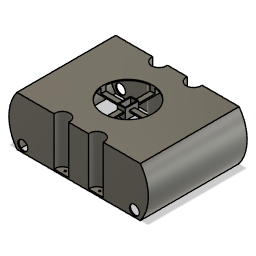
Carter (Autodesk Fusion 360 design; units mm, degrees)
Autodesk Fusion 360 part; units mm, degrees
sketch "Sketch1" plane through (0, 0, 0) normal (0, 0, 1) x (1, 0, 0)
  line L0 (0, 0) -> (-125, 0)
  line L1 (-125, 100) -> (0, 100)
  line L2 (0, 100) -> (0, 0)
  arc A0 (-125, 100) -> (-125, 0) centre (-56.2614, 50) ccw
  arc A1 (-124.4112, 98) -> (-123, 0) centre (-54.2614, 50) ccw
  line L3 (0, 98) -> (-124.4112, 98)
  line L4 (-175, 98) -> (-175, -10)
  line L5 (-175, -10) -> (191.1619, -10)
  line L6 (191.1619, -10) -> (191.1619, 126.0853)
  line L7 (191.1619, 126.0853) -> (-175, 126.0853)
  line L8 (-175, 126.0853) -> (-175, 98)
  line L9 (0, 98) -> (124.4112, 98)
  line L10 (125, 100) -> (0, 100)
  arc A2 (123, 0) -> (124.4112, 98) centre (54.2614, 50) ccw
  arc A3 (125, 0) -> (125, 100) centre (56.2614, 50) ccw
  line L11 (0, 0) -> (125, 0)
  circle A4 centre (113, 12.5) radius 10
  circle A5 centre (-113, 12.5) radius 10
  dimension "d1" = 125
  dimension "d2" = 100
  dimension "d3" = 85
  dimension "d4" = 85
  dimension "d6" = 2
  dimension "d7" = 2
  dimension "d44" = 20
  dimension "d45" = 12
  dimension "d46" = 12.5
  constraint horizontal L0
  constraint horizontal L1
  constraint vertical L2
  constraint coincident L0.start L2.end
  constraint coincident L0 A1.end
  constraint coincident L2 L3.start
  constraint perpendicular L2 L3
  constraint perpendicular L3 L4
  constraint perpendicular L4 L5
  constraint perpendicular L5 L6
  constraint perpendicular L6 L7
  constraint perpendicular L3 L8
  constraint symmetric L0.start L2 L11.start
  constraint symmetric L0.end L2 A3.start
  constraint symmetric L1.start L2 L10.start
  constraint symmetric L1.end L2 L10.end
  constraint symmetric L2 A0 A3
  constraint symmetric L2 A1.end A2.start
  constraint symmetric L2 A1 A2
  constraint symmetric L2 L3.start L9.start
  constraint symmetric L2 A1.start L9.end
  constraint symmetric L2 A4 A5
  measures "d1" distance of L0.start L0.end
  measures "d2" distance of L0.start L1.end
  measures "d3" radius of A0
  measures "d4" radius of A1
  measures "d6" distance of L0.end A1.end
  measures "d7" distance of L1 L3
  measures "d44" diameter of A4
  measures "d45" horizontal distance of A3.start A4.centre
  measures "d46" distance of L11 A4.centre
extrude "Extrude1" add sketch "Sketch1" along normal blind 196 contours L0 L1 L2 A0 A1 L3 | L2 L9 L10 A2 A3 L11 makes body 1
sketch "Sketch2" plane through (0, 100, 0) normal (0, 1, 0) x (-1, 0, 0)
  line L0 (-125, 0) -> (125, 0)
  line L1 (125, 0) -> (125, 196)
  line L2 (125, 196) -> (-125, 196)
  line L3 (-125, 196) -> (-125, 0)
  line L4 (56.5763, 0) -> (165.4437, 0)
  line L5 (165.4437, 0) -> (165.4437, -2)
  line L6 (165.4437, -2) -> (56.5763, -2)
  line L7 (56.5763, -2.1497) -> (56.5763, -2)
  line L8 (27.1632, 196) -> (155, 196)
  line L9 (155, 196) -> (155, 198)
  line L10 (155, 198) -> (27.1632, 198)
  line L11 (27.1632, 196) -> (-160, 196)
  line L12 (-160, 196) -> (-160, 198)
  line L13 (-160, 198) -> (27.1632, 198)
  line L14 (56.5763, 0) -> (-160, 0)
  line L15 (-160, 0) -> (-160, -2)
  line L16 (-160, -2) -> (56.5763, -2)
  line L17 (56.5763, -2) -> (56.5763, 0)
  circle A0 centre (-35, 196) radius 15
  circle A1 centre (-35, 196) radius 17
  circle A2 centre (35, 196) radius 15
  circle A3 centre (35, 196) radius 17
  circle A4 centre (-35, 0) radius 17
  circle A5 centre (-35, 0) radius 15
  circle A6 centre (35, 0) radius 17
  circle A7 centre (35, 0) radius 15
  circle A8 centre (-35, 6) radius 2
  circle A9 centre (35, 6) radius 2
  line L18 (-50, 0) -> (-50, 25)
  line L19 (20, 0) -> (20, 24.2158)
  circle A10 centre (35, 190) radius 2
  circle A11 centre (-35, 190) radius 2
  circle A12 centre (0, 98) radius 50
  line L20 (65, 103) -> (65, 93)
  line L21 (-65, 93) -> (-65, 103)
  line L22 (-5, 33) -> (5, 33)
  line L23 (5, 163) -> (-5, 163)
  line L24 (-6, 109.5) -> (6, 109.5)
  line L25 (6, 86.5) -> (-6, 86.5)
  line L26 (-8, 93) -> (-65, 93)
  line L27 (65, 93) -> (8, 93)
  line L28 (5, 33) -> (5, 84.5)
  line L29 (5, 111.5) -> (5, 163)
  line L30 (65, 103) -> (8, 98.6154) construction
  line L31 (-8, 97.3846) -> (-65, 93) construction
  line L32 (-65, 103) -> (-8, 98.6154) construction
  line L33 (8, 97.3846) -> (65, 93) construction
  line L34 (-125, 98) -> (-8, 98)
  line L35 (8, 98) -> (125, 98)
  line L36 (-5, 33) -> (-1.0385, 84.5) construction
  line L37 (1.0385, 111.5) -> (5, 163) construction
  line L38 (5, 33) -> (1.0385, 84.5) construction
  line L39 (-1.0385, 111.5) -> (-5, 163) construction
  line L40 (-65, 103) -> (-8, 103)
  line L41 (8, 103) -> (65, 103)
  line L42 (-5, 84.5) -> (-5, 33)
  line L43 (-5, 163) -> (-5, 111.5)
  line L44 (6, 109.5) -> (6, 98)
  line L45 (6, 97.5385) -> (6, 86.5)
  line L46 (-6, 86.5) -> (-6, 98.4615)
  line L47 (-6, 103) -> (-6, 109.5)
  line L48 (-6, 103) -> (-6, 98.4615)
  line L49 (-8, 84.5) -> (8, 84.5)
  line L50 (8, 84.5) -> (8, 111.5)
  line L51 (8, 111.5) -> (-8, 111.5)
  line L52 (-8, 111.5) -> (-8, 84.5)
  line L53 (6, 98) -> (6, 97.5385)
  point P0 (0, 98)
  point P1 (0, 98)
  point P2 (0, 98)
  point P3 (0, 98)
  dimension "d10" = 2
  dimension "d11" = 2
  dimension "d12" = 2
  dimension "d15" = 2
  dimension "d22" = 30
  dimension "d23" = 34
  dimension "d24" = 30
  dimension "d25" = 34
  dimension "d26" = 90
  dimension "d27" = 90
  dimension "d35" = 4
  dimension "d36" = 4
  dimension "d37" = 15
  dimension "d38" = 15
  dimension "d39" = 6
  dimension "d40" = 6
  dimension "d41" = 100
  dimension "d55" = 130
  dimension "d56" = 10
  dimension "d57" = 10
  dimension "d58" = 130
  dimension "d59" = 12
  dimension "d60" = 23
  dimension "d61" = 16
  dimension "d62" = 27
  constraint perpendicular L4 L5
  constraint parallel L4 L6
  constraint perpendicular L1 L4
  constraint coincident L0 L4.start
  constraint vertical L7
  constraint horizontal L8
  constraint vertical L9
  constraint horizontal L10
  constraint coincident L2 L8.start
  constraint horizontal L11
  constraint vertical L12
  constraint horizontal L13
  constraint horizontal L14
  constraint vertical L15
  constraint horizontal L16
  constraint vertical L17
  constraint concentric A0 A1
  constraint concentric A2 A3
  constraint midpoint L3 L34.start
  constraint midpoint L1 L35.end
  constraint coincident L8 A2.centre
  constraint coincident L11 A0.centre
  constraint symmetric A0 A5 L34
  constraint symmetric A1 A4 L34
  constraint symmetric A2 A7 L34
  constraint symmetric A3 A6 L34
  constraint coincident A5 L18.start
  constraint coincident L14 L18.start
  constraint tangent A5 L18
  constraint coincident A7 L19.start
  constraint coincident L14 L19.start
  constraint tangent A7 L19
  constraint symmetric A8 A11 L34
  constraint symmetric A9 A10 L34
  constraint horizontal L40
  constraint perpendicular L20 L40
  constraint parallel L27 L40
  constraint parallel L20 L21
  constraint coincident P3 L32
  constraint coincident P3 L30
  constraint coincident P3 P2
  constraint horizontal L22
  constraint perpendicular L22 L28
  constraint parallel L22 L23
  constraint parallel L28 L43
  constraint coincident P3 L36
  constraint coincident P3 L38
  constraint horizontal L24
  constraint perpendicular L24 L44
  constraint parallel L24 L25
  constraint parallel L44 L46
  constraint collinear L26 L27
  constraint collinear L30 L31
  constraint collinear L32 L33
  constraint collinear L34 L35
  constraint collinear L36 L37
  constraint collinear L38 L39
  constraint collinear L40 L41
  constraint collinear L42 L43
  constraint coincident L47.start L46
  constraint coincident L45.start L44
  constraint collinear L44 L45
  constraint collinear L46 L47
  constraint horizontal L49
  constraint perpendicular L49 L50
  constraint parallel L49 L51
  constraint parallel L50 L52
  constraint coincident L49 L28.end
  constraint coincident L50 L27.end
  constraint coincident L50 L35.start
  constraint coincident L50 L33.start
  constraint coincident L50 L30.end
  constraint coincident L50 L41.start
  constraint coincident L52 L34.end
  constraint coincident L52 L32.end
  constraint coincident L52 L31.start
  constraint coincident L52 L26.start
  constraint coincident L49 L42.start
  constraint coincident L49 L36.end
  constraint coincident L49 L38.end
  constraint coincident L52 L40.end
  constraint coincident L51 L43.end
  constraint coincident L51 L29.start
  constraint coincident L51 L37.start
  constraint coincident L51 L39.start
  measures "d10" distance of L8 L10
  measures "d11" distance of L11 L13
  measures "d12" distance of L4 L6
  measures "d15" distance of L4.start L6.end
  measures "d22" diameter of A0
  measures "d23" diameter of A1
  measures "d24" diameter of A2
  measures "d25" diameter of A3
  measures "d26" distance of L3 A0.centre
  measures "d27" distance of L1 A2.centre
  measures "d35" diameter of A8
  measures "d36" diameter of A9
  measures "d37" distance of A8.centre L18
  measures "d38" distance of A9.centre L19
  measures "d39" distance of L14 A8.centre
  measures "d40" distance of L14 A9.centre
  measures "d41" diameter of A12
  measures "d55" distance of L20.end L21.start
  measures "d56" distance of L27 L40
  measures "d57" distance of L23.start L23.end
  measures "d58" distance of L22.end L23.start
  measures "d59" distance of L25.start L25.end
  measures "d60" distance of L24.end L25.start
  measures "d61" distance of L50.end L51.end
  measures "d62" distance of L49.end L50.end
extrude "Extrude2" add sketch "Sketch2" against normal blind 100 contours L0 L14 L16 A4 A5 | L0 L14 L16 A5 | L0 L14 L16 A4 A5 | L0 L14 L15 L16 A4 | L0 L14 L16 A4 A6 | L0 L14 L16 A6 A7 | L0 L14 L16 A7 | L2 L11 L12 L13 A1 | L0 L14 L16 A6 A7 | L0 L14 L16 L17 A6 | L2 L11 L13 A0 A1 | L0 L4 L5 L6 L17 | L2 L11 L13 A0 | L2 L11 L13 A1 A3 | L2 L11 L13 A0 A1 | L2 L11 L13 A2 A3 | L2 L8 L10 L11 L13 A2 | L2 L8 L9 L10 A3 | L2 L8 L10 A2 A3 bodies 1
extrude "Extrude3" cut sketch "Sketch1" along normal blind 270 and the other way blind 120 contours L4 L5 L6 L7 L8 bodies 1
extrude "Extrude4" cut sketch "Sketch2" against normal blind 120 contours L0 L14 A5 | L0 L14 L16 A5 | L0 L14 A7 | L0 L14 L16 A7 | L2 L11 L13 A0 | L2 L11 A0 | L2 L8 L10 L11 L13 A2 | L2 L8 L11 A2 | A8 | A9 | A10 | A11 bodies 1
extrude "Extrude5" add sketch "Sketch2" against normal blind 100 contours L0 L14 L16 A4 A5 | L0 L14 A4 A5 L18 | L0 L14 A4 L18 | L0 L14 L16 A4 A5 | L0 L14 A6 L19 | L0 L14 L16 A6 A7 | L0 L14 A6 A7 L19 | L0 L14 L16 A6 A7 | L2 L11 L13 A0 A1 | L2 L11 A0 A1 | L2 L11 L13 A0 A1 | L2 L11 L13 A2 A3 | L2 L8 L11 A2 A3 | L2 L8 L10 A2 A3 bodies 1
extrude "Extrude6" add sketch "Sketch2" against normal blind 3 from surface at -97 contours L0 L14 A5 | L0 L14 L16 A5 | L0 L14 A7 | L0 L14 L16 A7 | L2 L11 L13 A0 | L2 L11 A0 | L2 L8 L10 L11 L13 A2 | L2 L8 L11 A2 | A8 | A9 | A10 | A11 bodies 1
extrude "Extrude7" cut sketch "Sketch2" against normal blind 180 contours A12 L26 L34 L52 | A12 L34 L40 L52 | A12 L26 L42 L49 L52 | A12 L40 L43 L51 L52 | L49 L50 L51 L52 | A12 L28 L42 L49 | A12 L29 L43 L51 | A12 L27 L28 L49 L50 | A12 L29 L41 L50 L51 | A12 L27 L35 L50 | A12 L35 L41 L50 | A8 | A9 | A10 | A11 | L24 L25 L44 L45 L46 L47 L48 L53 bodies 1
extrude "Extrude8" cut sketch "Sketch1" along normal blind 250 and the other way blind 25 contours A4 | A5 bodies 1
extrude "Extrude9" add sketch "Sketch2" against normal blind 3 from surface at -12.5 separate body contours A12 L26 L34 L52 | A12 L34 L40 L52 | A12 L28 L42 L49 | A12 L29 L43 L51 | A12 L27 L35 L50 | A12 L35 L41 L50 makes body 2 at (0.5564, 87.5, 123.6574) makes body 3 at (21.9907, 84.5, 98.5564) makes body 4 at (-21.9907, 84.5, 98.5564) makes body 5 at (0.5564, 87.5, 72.3426)
extrude "Extrude10" add sketch "Sketch2" against normal blind 21.5 from surface at -5 contours L49 L50 L51 L52 bodies 2 3 4 5
extrude "Extrude11" add sketch "Sketch2" against normal blind 2 from surface at -24.5 contours L24 L25 L44 L45 L46 L47 L48 L53 bodies 2
extrude "Extrude12" add sketch "Sketch2" against normal blind 15.5 contours A12 L21 L26 L34 | A12 L21 L34 L40 | A12 L22 L28 L42 | A12 L23 L29 L43 | A12 L20 L35 L41 | A12 L20 L27 L35 bodies 1 2
sketch "Sketch3" plane through (0, 0, 86.5) normal (0, 0, 1) x (1, 0, 0)
  line L0 (-6, 75.5) -> (6, 75.5)
  line L1 (6, 75.5) -> (6, 95)
  line L2 (6, 95) -> (-6, 95)
  line L3 (-6, 95) -> (-6, 75.5)
  line L4 (-5, 77) -> (5, 77)
  line L5 (5, 77) -> (5, 84.4286)
  line L6 (5, 84.4286) -> (-5, 84.4286)
  line L7 (-5, 84.4286) -> (-5, 77)
  constraint horizontal L4
  constraint vertical L5
  constraint horizontal L6
  constraint vertical L7
extrude "Extrude13" cut sketch "Sketch3" against normal blind 2 contours L4 L5 L6 L7 bodies 1
